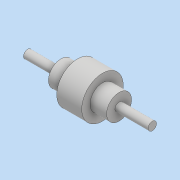
# Autodesk Inventor part: P1
Saved by Autodesk Inventor 2017 (Build 210142000, 142)
## iProperties
Part Number: P1
Material: 一般
Document SubType Name: Modeling
Designer: d8910
Density: 1 g/cm^3
Appearance: 預設
Author: d8910
Autodesk Inventor part; units mm, degrees
ref_plane "YZ Plane" through (0, 0, 0) normal (1, 0, 0) x (0, 1, 0)
ref_plane "XZ Plane" through (0, 0, 0) normal (0, 1, 0) x (-1, 0, 0)
ref_plane "XY Plane" through (0, 0, 0) normal (0, 0, 1) x (1, 0, 0)
sketch "草圖1" plane through (0, 0, 0) normal (0, 0, 1) x (1, 0, 0)
  line L0 (0, 0) -> (-30, 0)
  line L1 (-30, 0) -> (-30, 50)
  line L2 (-30, 50) -> (0, 50)
  line L3 (0, 50) -> (0, 0)
  line L4 (-30, 0) -> (-70, 0)
  line L5 (-70, 0) -> (-70, 30)
  line L6 (-70, 30) -> (-30, 30)
  line L7 (-30, 30) -> (-30, 0)
  line L8 (-70, 0) -> (-150, 0)
  line L9 (-150, 0) -> (-150, 10)
  line L10 (-150, 10) -> (-70, 10)
  line L11 (-70, 10) -> (-70, 0)
  dimension "d0" = 30
  dimension "d1" = 40
  dimension "d2" = 80
  dimension "d3" = 10
  dimension "d4" = 30
  dimension "d5" = 50
  constraints: 24 end point, 6 parallel, 3 horizontal, 3 perpendicular
  measures "d0" distance of L1.end L2.end
  measures "d1" distance of L5.end L6.end
  measures "d2" distance of L9.end L10.end
  measures "d3" distance of L8.end L9.end
  measures "d4" distance between parallel lines of L4 L6
  measures "d5" distance between parallel lines of L0 L2
revolve "迴轉1" add sketch "草圖1" angle 360 about axis through (-70, 0, 0) along (-1, 0, 0)
mirror "鏡射1" about plane through (0, 0, 0) normal (1, 0, 0) of "迴轉1"
